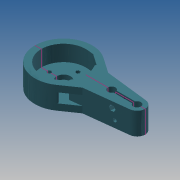
# Autodesk Inventor part: distal arm
Saved by Autodesk Inventor 2013 (Build 170138000, 138)
## iProperties
Created: 2017-03-30
Part Number: distal arm
Material: Generic
Document SubType Name: Modeling
Designer: employee
Density: 1 g/cm^3
Author: employee
Autodesk Inventor part; units mm, degrees
ref_plane "YZ Plane" through (0, 0, 0) normal (1, 0, 0) x (0, 1, 0)
ref_plane "XZ Plane" through (0, 0, 0) normal (0, 1, 0) x (-1, 0, 0)
ref_plane "XY Plane" through (0, 0, 0) normal (0, 0, 1) x (1, 0, 0)
sketch "Sketch1" plane through (0, 0, 0) normal (0, 0, 1) x (1, 0, 0)
  arc A0 (43.229, 12.5) -> (43.229, -12.5) centre (0, 0) ccw
  line L0 (0, 12.5) -> (115.5, 12.5)
  arc A1 (115.5, -12.5) -> (115.5, 12.5) centre (115.5, 0) ccw
  line L1 (115.5, -12.5) -> (0, -12.5)
  arc A2 (0, 12.5) -> (0, -12.5) centre (0, 0) ccw
  circle A3 centre (115.5, 0) radius 6
  circle A4 centre (75.5, 0) radius 6.0311
  dimension "d0" = 90
  dimension "d2" = 25
  dimension "d3" = 115.5
  dimension "d4" = 12
  dimension "d5" = 12.0622
  dimension "d6" = 40
  constraints: 6 point on circle, 5 centre point, 4 end point, 4 tangent, 3 coincident, 2 point on line, 1 horizontal, 1 horizontal alignment, 1 parallel
  measures "d0" diameter of A0
  measures "d2" distance between parallel lines of L0 L1
  measures "d3" distance of L1.start L1.end
  measures "d4" diameter of A3
  measures "d5" diameter of A4
  measures "d6" distance of A1.centre A4.centre
extrude "Extrusion1" add sketch "Sketch1" along normal blind 35
sketch "Sketch2" plane through (0, 0, 35) normal (0, 0, 1) x (1, 0, 0)
  arc A0 (43.229, 12.5) -> (43.229, -12.5) centre (0, 0) ccw projected
  circle A1 centre (0, 0) radius 35
  dimension "d9" = 10
  constraints: 1 centre point, 1 coincident
  measures "d9" radial gap between concentric circles of A0 A1
extrude "Extrusion2" cut sketch "Sketch2" against normal blind 25
sketch "Sketch3" plane through (0, 0, 0) normal (0, 0, -1) x (-1, 0, 0)
  arc A0 (-43.229, -12.5) -> (-43.229, 12.5) centre (0, 0) ccw projected
  circle A1 centre (0, 22.5) radius 1.75
  circle A2 centre (0, 40) radius 1.75
  dimension "d12" = 22.5
  dimension "d13" = 3.5
  dimension "d30" = 40
  constraints: 2 centre point, 2 vertical alignment, 1 equal radius
  measures "d12" distance of A1.centre A0.centre
  measures "d13" diameter of A1
  measures "d30" distance of A2.centre A0.centre
extrude "Extrusion3" cut sketch "Sketch3" against normal through all contours A1
sketch "Sketch4" plane through (0, 0, 10) normal (0, 0, 1) x (1, 0, 0)
  circle A0 centre (0, 22.5) radius 1.75 projected
  line L0 (3.1754, 22.5) -> (1.5877, 19.75)
  line L1 (1.5877, 19.75) -> (-1.5877, 19.75)
  line L2 (-1.5877, 19.75) -> (-3.1754, 22.5)
  line L3 (-3.1754, 22.5) -> (-1.5877, 25.25)
  line L4 (-1.5877, 25.25) -> (1.5877, 25.25)
  line L5 (1.5877, 25.25) -> (3.1754, 22.5)
  dimension "d16" = 5.5
  constraints: 12 end point, 1 coincident, 1 horizontal, 13 other
  measures "d16" distance between parallel lines of L1 L4
extrude "Extrusion4" cut sketch "Sketch4" against normal blind 4
pattern_circular "Circular Pattern1" count 4 over 360 about axis through (0, 0, 35) along (0, 0, -1) of "Extrusion4", "Extrusion3"
sketch "Sketch5" plane through (0, 0, 10) normal (0, 0, 1) x (1, 0, 0)
  circle A0 centre (0, 0) radius 35 projected
  circle A1 centre (0, 0) radius 7.5
  dimension "d22" = 15
  constraints: 1 centre point, 1 coincident
  measures "d22" diameter of A1
extrude "Extrusion5" cut sketch "Sketch5" against normal through all contours A1
sketch "Sketch6" plane through (0, 0, 10) normal (0, 0, 1) x (1, 0, 0)
  circle A0 centre (0, 0) radius 7.5 projected
  circle A1 centre (0, 0) radius 35 projected
  circle A2 centre (0, 0) radius 11
  dimension "d26" = 22
  constraints: 1 centre point, 1 coincident
  measures "d26" diameter of A2
extrude "Extrusion6" cut sketch "Sketch6" against normal blind 7 contours A2
sketch "Sketch13" plane through (0, 0, 35) normal (0, 0, 1) x (1, 0, 0)
  line L0 (43.229, -12.5) -> (115.5, -12.5) projected
  arc A0 (115.5, -12.5) -> (115.5, 12.5) centre (115.5, 0) ccw projected
  arc A1 (43.229, 12.5) -> (43.229, -12.5) centre (0, 0) ccw projected
  circle A2 centre (0, 0) radius 31.831
  line L1 (3.6739, -31.6183) -> (168.2078, -12.5)
  line L2 (116.9428, -12.4165) -> (39.5829, -21.4054)
  dimension "d67" = 63.662
  dimension "d69" = 6
  constraints: 4 end point, 2 point on circle, 1 coincident, 1 parallel, 1 point on line, 1 tangent, 4 other
  measures "d69" distance between parallel lines of L2 L1
extrude "Extrusion13" add sketch "Sketch13" against normal up to surface (35 mm away) contours L0 A0 L2 A1
sketch "Sketch14" plane through (0, 0, 0) normal (0, 1, 0) x (-1, 0, 0)
  line L0 (19.75, 10) -> (19.75, 6) projected
  line L1 (19.75, 6) -> (20.75, 6) projected
  line L2 (20.75, 6) -> (20.75, 0) projected
  line L3 (20.75, 0) -> (7.5, 0) projected
  line L4 (7.5, 0) -> (7.5, 3) projected
  line L5 (7.5, 3) -> (11, 3) projected
  line L6 (11, 3) -> (11, 10) projected
  line L7 (11, 10) -> (19.75, 10) projected
  line L8 (35, 35) -> (45, 35) projected
  line L9 (45, 35) -> (45, 0) projected
  line L10 (45, 0) -> (24.25, 0) projected
  line L11 (-19.75, 6) -> (-19.75, 10) projected
  line L12 (-19.75, 10) -> (-11, 10) projected
  line L13 (-11, 10) -> (-11, 3) projected
  line L14 (-11, 3) -> (-7.5, 3) projected
  line L15 (-7.5, 3) -> (-7.5, 0) projected
  line L16 (-7.5, 0) -> (-20.75, 0) projected
  line L17 (-20.75, 0) -> (-20.75, 6) projected
  line L18 (-20.75, 6) -> (-19.75, 6) projected
  line L19 (35, 10) -> (35, 35) projected
  line L20 (24.25, 0) -> (24.25, 6) projected
  line L21 (24.25, 6) -> (25.25, 6) projected
  line L22 (25.25, 6) -> (25.25, 10) projected
  line L23 (25.25, 10) -> (35, 10) projected
  line L24 (-35, 35) -> (-35, 10) projected
  line L25 (-35, 10) -> (-25.25, 10) projected
  line L26 (-25.25, 10) -> (-25.25, 6) projected
  line L27 (-25.25, 6) -> (-24.25, 6) projected
  line L28 (-24.25, 6) -> (-24.25, 0) projected
  line L29 (-24.25, 0) -> (-69.4689, 0) projected
  line L30 (-69.4689, 35) -> (-35, 35) projected
  line L31 (-69.4689, 0) -> (-69.4689, 35) projected
  line L32 (-109.5, 0) -> (-109.5, 35) projected
  line L33 (-109.5, 35) -> (-81.5311, 35) projected
  line L34 (-81.5311, 35) -> (-81.5311, 0) projected
  line L35 (-81.5311, 0) -> (-109.5, 0) projected
  line L36 (-121.5, 35) -> (-121.5, 0) projected
  line L37 (-121.5, 0) -> (-128, 0) projected
  line L38 (-128, 0) -> (-128, 35) projected
  line L39 (-128, 35) -> (-121.5, 35) projected
  line L40 (-95.5155, 35) -> (-95.5155, 0)
  point P0 (0, 0)
  constraints: 2 end point, 2 midpoint
mirror "Mirror1" about plane through (0, 0, 0) normal (0, 1, 0) of "Extrusion13"
sketch "Sketch16" plane through (116.9428, -12.4165, 0) normal (0.11542, -0.9933168, 0) x (0.9933168, 0.11542, 0)
  line L0 (0, 0) -> (-77.8803, 0) projected
  line L1 (-19.8509, 35) -> (-19.8509, 0) projected
  circle A0 centre (-21.8509, 10.725) radius 2.75
  point P0 (-114.7281, 0)
  point P1 (-19.8061, 35)
  point P2 (-19.8061, 0)
  dimension "d72" = 10.725
  dimension "d73" = 5.5
  dimension "d94" = 2
  constraints: 1 centre point, 1 other
  measures "d72" distance from line of A0.centre L0
  measures "d73" diameter of A0
extrude "Extrusion14" cut sketch "Sketch16" against normal blind 29
sketch "Sketch17" plane through (39.5829, 21.4054, 35) normal (0.11542, 0.9933168, 0) x (0.9933168, -0.11542, 0)
  line L0 (77.8803, 35) -> (0, 35) projected
  line L1 (58.0294, 0) -> (58.0294, 35) projected
  circle A0 centre (56.0294, 9.525) radius 2.75
  point P0 (-36.8478, 35)
  point P1 (42.4536, 0)
  point P2 (42.4536, 35)
  dimension "d76" = 25.475
  dimension "d77" = 5.5
  dimension "d107" = 2
  constraints: 1 centre point, 1 other
  measures "d76" distance from line of A0.centre L0
  measures "d77" diameter of A0
extrude "Extrusion15" cut sketch "Sketch17" against normal blind 29
sketch "Sketch18" plane through (91.8907, 13.8677, 10.725) normal (0.11542, -0.9933168, 0) x (0.9933168, 0.11542, 0)
  circle A0 centre (0, 0) radius 2.75 projected
  line L0 (4.6188, 0) -> (2.3094, -4)
  line L1 (2.3094, -4) -> (-2.3094, -4)
  line L2 (-2.3094, -4) -> (-4.6188, 0)
  line L3 (-4.6188, 0) -> (-2.3094, 4)
  line L4 (-2.3094, 4) -> (2.3094, 4)
  line L5 (2.3094, 4) -> (4.6188, 0)
  point P0 (-92.8772, -10.725)
  dimension "d80" = 8
  constraints: 12 end point, 1 coincident, 1 horizontal, 13 other
  measures "d80" distance between parallel lines of L1 L4
extrude "Extrusion16" cut sketch "Sketch18" against normal blind 10000 and the other way blind 5 contours A0 | L0 L1 L2 L3 L4 L5
sketch "Sketch19" plane through (91.8907, -13.8677, 25.475) normal (0.11542, 0.9933168, 0) x (0.9933168, -0.11542, 0)
  circle A0 centre (0, 0) radius 2.75 projected
  line L0 (-4.6188, 0) -> (-2.3094, 4)
  line L1 (-2.3094, 4) -> (2.3094, 4)
  line L2 (2.3094, 4) -> (4.6188, 0)
  line L3 (4.6188, 0) -> (2.3094, -4)
  line L4 (2.3094, -4) -> (-2.3094, -4)
  line L5 (-2.3094, -4) -> (-4.6188, 0)
  point P0 (-92.8772, 25.475)
  dimension "d85" = 8
  constraints: 12 end point, 1 coincident, 1 horizontal, 13 other
  measures "d85" distance between parallel lines of L4 L1
extrude "Extrusion17" cut sketch "Sketch19" against normal blind 10000 and the other way blind 5 contours A0 | L0 L1 L2 L3 L4 L5
sketch "Sketch20" plane through (0, 0, 35) normal (0, 0, 1) x (1, 0, 0)
  circle A0 centre (75.5, 0) radius 6.0311 projected
  circle A1 centre (115.5, 0) radius 6 projected
  line L0 (75.5, 2.5) -> (115.5, 2.5)
  line L1 (115.5, 2.5) -> (115.5, -2.5)
  line L2 (115.5, -2.5) -> (75.5, -2.5)
  line L3 (75.5, -2.5) -> (75.5, 2.5)
  dimension "d90" = 5
  constraints: 8 end point, 2 coincident, 2 midpoint, 2 parallel, 1 horizontal, 1 perpendicular
  measures "d90" distance between parallel lines of L2 L0
extrude "Extrusion18" cut sketch "Sketch20" against normal through all contours A0 L2 L3 L0 | A0 L0 A1 L2 | L0 L1 L2 A1 picked at (77.5104, 0) picked at (113.5, 0)
sketch "Sketch21" plane through (0, 0, 35) normal (0, 0, 1) x (1, 0, 0)
  circle A0 centre (0, 0) radius 35 construction
  line L0 (39.5829, 21.4054) -> (116.9428, 12.4165) construction
  line L1 (39.5829, -21.4054) -> (116.9428, -12.4165) projected
  line L2 (39.5829, -21.4054) -> (2.9814, -25.6584)
  line L3 (2.9814, -25.6584) -> (4.0397, -34.7661)
  line L4 (4.0397, -34.7661) -> (40.6412, -30.5131)
  line L5 (40.6412, -30.5131) -> (39.5829, -21.4054)
  line L6 (39.5829, 21.4054) -> (2.9814, 25.6584)
  line L7 (2.9814, 25.6584) -> (4.0397, 34.7661)
  line L8 (4.0397, 34.7661) -> (40.6412, 30.5131)
  line L9 (40.6412, 30.5131) -> (39.5829, 21.4054)
  constraints: 16 end point, 4 parallel, 2 collinear, 2 perpendicular, 2 point on circle, 2 tangent
extrude "Extrusion19" cut sketch "Sketch21" against normal up to surface (25 mm away)
fillet "Fillet2" radius 2.5 4 edges at (26.4405, 22.9325, 22.5) (32.1349, 31.5015, 22.5) (26.4405, -22.9325, 22.5) (32.1349, -31.5015, 22.5)
sketch "Sketch23" plane through (0, 0, 35) normal (0, 0, 1) x (1, 0, 0)
  line L0 (4.0397, 34.7661) -> (23.906, 32.4577) projected
  arc A0 (23.906, 32.4577) -> (25.6178, 36.9963) centre (24.1946, 34.941) ccw projected
  arc A1 (25.6178, 36.9963) -> (25.6178, -36.9963) centre (0, 0) ccw projected
  line L1 (110.0456, -2.5) -> (80.9885, -2.5) projected
  arc A2 (80.9885, 2.5) -> (80.9885, -2.5) centre (75.5, 0) ccw projected
  line L2 (80.9885, 2.5) -> (110.0456, 2.5) projected
  arc A3 (110.0456, -2.5) -> (110.0456, 2.5) centre (115.5, 0) ccw projected
  arc A4 (29.7314, -18.4674) -> (32.1436, -22.2698) centre (31.855, -19.7865) ccw projected
  line L3 (32.1436, -22.2698) -> (116.9428, -12.4165) projected
  arc A5 (116.9428, -12.4165) -> (116.9428, 12.4165) centre (115.5, 0) ccw projected
  line L4 (116.9428, 12.4165) -> (32.1436, 22.2698) projected
  arc A6 (32.1436, 22.2698) -> (29.7314, 18.4674) centre (31.855, 19.7865) ccw projected
  arc A7 (29.7314, -18.4674) -> (29.7314, 18.4674) centre (0, 0) ccw projected
  line L5 (25.6178, 36.9963) -> (49.8579, 20.2115)
  line L6 (12.7312, 33.7562) -> (30.1999, 21.6602)
  dimension "d102" = 10
  constraints: 4 end point, 2 point on line, 2 tangent, 1 parallel, 1 point on circle
  measures "d102" distance between parallel lines of L5 L6
extrude "Extrusion21" add sketch "Sketch23" against normal blind 10 contours L0 A0 L5 L4 A6 L6
mirror "Mirror2" about plane through (0, 0, 0) normal (0, 1, 0) of "Extrusion21"
sketch "Sketch24" plane through (0, 0, 0) normal (0, 0, -1) x (-1, 0, 0)
  line L0 (-23.906, 32.4577) -> (-12.7312, 33.7562) projected
  arc A0 (-25.6178, 36.9963) -> (-23.906, 32.4577) centre (-24.1946, 34.941) ccw projected
  line L1 (-25.6178, 36.9963) -> (-49.8579, 20.2115) projected
  line L2 (-32.1436, 22.2698) -> (-49.8579, 20.2115) projected
  arc A1 (-30.1999, 21.6602) -> (-32.1436, 22.2698) centre (-31.855, 19.7865) ccw projected
  line L3 (-30.1999, 21.6602) -> (-12.7312, 33.7562) projected
  line L4 (-12.7312, -33.7562) -> (-23.906, -32.4577) projected
  line L5 (-30.1999, -21.6602) -> (-12.7312, -33.7562) projected
  arc A2 (-32.1436, -22.2698) -> (-30.1999, -21.6602) centre (-31.855, -19.7865) ccw projected
  line L6 (-49.8579, -20.2115) -> (-32.1436, -22.2698) projected
  line L7 (-25.6178, -36.9963) -> (-49.8579, -20.2115) projected
  arc A3 (-23.906, -32.4577) -> (-25.6178, -36.9963) centre (-24.1946, -34.941) ccw projected
extrude "Extrusion22" add sketch "Sketch24" against normal up to surface (10 mm away)
sketch "Sketch8" plane through (43.229, 12.5, 0) normal (0, 1, 0) x (1, 0, 0)
  line L0 (72.271, -35) -> (0, -35) projected
  line L1 (72.271, 0) -> (72.271, -35) projected
  line L2 (38.302, 0) -> (38.302, -35) projected
  line L3 (26.2399, 0) -> (26.2399, -35) projected
  line L4 (26.2399, -17.5) -> (38.302, -17.5)
  line L5 (32.271, -17.5) -> (72.271, -17.5)
  circle A0 centre (52.271, -28.5) radius 2.75
  circle A1 centre (52.271, -11.5) radius 2.75
  point P0 (-43.229, 0)
  point P1 (52.271, -17.5)
  dimension "d36" = 6.5
  dimension "d37" = 5.5
  dimension "d38" = 17
  constraints: 5 midpoint, 4 end point, 2 centre point, 2 vertical alignment, 1 equal radius
  measures "d36" distance from line of A0.centre L0
  measures "d37" diameter of A0
  measures "d38" distance of A1.centre A0.centre
sketch "Sketch9" plane through (43.229, 12.5, 0) normal (0, 1, 0) x (1, 0, 0)
  circle A0 centre (36.771, -28.5) radius 2.75 projected
  circle A1 centre (36.771, -28.5) radius 5
  point P0 (-43.229, 0)
  dimension "d41" = 10
  constraints: 1 centre point, 1 coincident
  measures "d41" diameter of A1
sketch "Sketch10" plane through (43.229, 12.5, 0) normal (0, 1, 0) x (1, 0, 0)
  arc A0 (39.3999, -10.693) -> (34.142, -10.693) centre (36.771, -11.5) ccw projected
  line L0 (34.4616, -7.5) -> (39.0804, -7.5)
  line L1 (39.0804, -7.5) -> (41.3898, -11.5)
  line L2 (41.3898, -11.5) -> (39.0804, -15.5)
  line L3 (39.0804, -15.5) -> (34.4616, -15.5)
  line L4 (34.4616, -15.5) -> (32.1522, -11.5)
  line L5 (32.1522, -11.5) -> (34.4616, -7.5)
  point P0 (-43.229, 0)
  dimension "d48" = 8
  constraints: 12 end point, 1 coincident, 1 horizontal, 13 other
  measures "d48" distance between parallel lines of L3 L0
sketch "Sketch11" plane through (43.229, -12.5, 0) normal (0, -1, 0) x (1, 0, 0)
  circle A0 centre (36.771, 11.5) radius 2.75 projected
  circle A1 centre (36.771, 11.5) radius 5
  point P0 (-43.229, 0)
  dimension "d53" = 10
  constraints: 1 centre point
  measures "d53" diameter of A1
sketch "Sketch12" plane through (43.229, -12.5, 35) normal (0, -1, 0) x (1, 0, 0)
  arc A0 (39.3999, -5.693) -> (34.142, -5.693) centre (36.771, -6.5) ccw projected
  line L0 (34.4616, -2.5) -> (39.0804, -2.5)
  line L1 (39.0804, -2.5) -> (41.3898, -6.5)
  line L2 (41.3898, -6.5) -> (39.0804, -10.5)
  line L3 (39.0804, -10.5) -> (34.4616, -10.5)
  line L4 (34.4616, -10.5) -> (32.1522, -6.5)
  line L5 (32.1522, -6.5) -> (34.4616, -2.5)
  point P0 (-43.229, -35)
  point P1 (36.771, -2.5)
  dimension "d60" = 8
  constraints: 12 end point, 1 coincident, 1 horizontal alignment, 1 midpoint, 13 other
  measures "d60" distance between parallel lines of L3 L0
body "Solid1"
